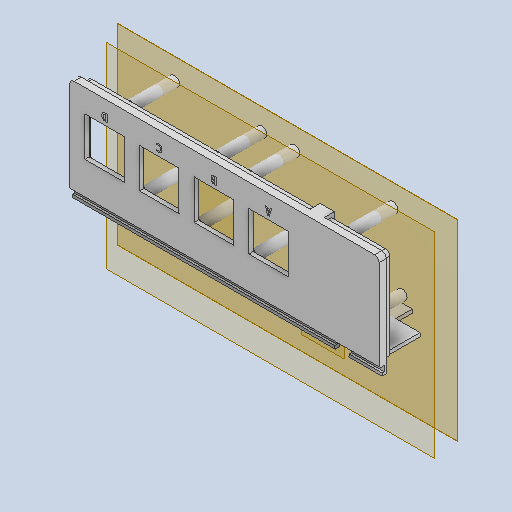
# Autodesk Inventor part: RV_ES_TopHV
Saved by Autodesk Inventor 2023.3 (Build 273359000, 359)
## iProperties
Created: 2023-08-06
Part Number: RV_ES_TopHV
Material: Generic
Document SubType Name: Modeling
Designer: atrus
Density: 1 g/cm^3
Appearance: Default
Author: atrus
Autodesk Inventor part; units mm, degrees
ref_plane "YZ Plane" through (0, 0, 0) normal (1, 0, 0) x (0, 1, 0)
ref_plane "XZ Plane" through (0, 0, 0) normal (0, 1, 0) x (-1, 0, 0)
ref_plane "XY Plane" through (0, 0, 0) normal (0, 0, 1) x (1, 0, 0)
ref_plane "Work Plane1" through (160.7185, -7.9424, -39.0916) normal (0, 0, 1) x (1, 0, 0)
ref_plane "Bottom Case Offset" through (160.7185, -7.9424, -38.8916) normal (0, 0, 1) x (1, 0, 0)
sketch "Sketch1" plane through (0, 0, 0) normal (0, 0, 1) x (1, 0, 0)
  line L0 (0, 55.6141) -> (215.9, 55.6141)
  line L1 (215.9, 55.6141) -> (215.9, 121.7246)
  line L2 (215.9, 121.7246) -> (0, 121.7246)
  line L3 (0, 121.7246) -> (0, 55.6141)
  line L4 (215.9, 121.7246) -> (215.9, 57.6563) construction
  line L5 (19.0355, 55.6141) -> (3.81, 55.6141) construction
  line L6 (0, 48.8987) -> (0, 118.5496) construction
  point P0 (0, 88.6694)
  constraints: 8 end point, 2 horizontal, 1 collinear, 1 midpoint, 1 parallel, 1 perpendicular, 1 point on line, 3 other
extrude "Top Face" add sketch "Sketch1" along normal blind 5
sketch "Sketch2" plane through (0, 0, 5) normal (0, 0, 1) x (1, 0, 0)
  line L0 (37.1761, 79.276) -> (11.6745, 79.276) construction
  line L1 (37.1761, 104.7776) -> (37.1761, 79.276) construction
  line L2 (11.6745, 104.7776) -> (37.1761, 104.7776) construction
  line L3 (11.6745, 79.276) -> (11.6745, 104.7776) construction
  line L4 (49.7745, 79.276) -> (49.7745, 104.7776) construction
  line L5 (49.7745, 104.7776) -> (75.2761, 104.7776) construction
  line L6 (75.2761, 104.7776) -> (75.2761, 79.276) construction
  line L7 (75.2761, 79.276) -> (49.7745, 79.276) construction
  line L8 (87.8745, 79.276) -> (87.8745, 104.7776) construction
  line L9 (87.8745, 104.7776) -> (113.3761, 104.7776) construction
  line L10 (113.3761, 104.7776) -> (113.3761, 79.276) construction
  line L11 (113.3761, 79.276) -> (87.8745, 79.276) construction
  line L12 (125.9745, 79.276) -> (125.9745, 104.7776) construction
  line L13 (125.9745, 104.7776) -> (151.4761, 104.7776) construction
  line L14 (151.4761, 104.7776) -> (151.4761, 79.276) construction
  line L15 (151.4761, 79.276) -> (125.9745, 79.276) construction
  line L16 (38.1761, 78.276) -> (10.6745, 78.276)
  line L17 (10.6745, 78.276) -> (10.6745, 105.7776)
  line L18 (10.6745, 105.7776) -> (38.1761, 105.7776)
  line L19 (38.1761, 105.7776) -> (38.1761, 78.276)
  line L20 (76.2761, 78.276) -> (76.2761, 105.7776)
  line L21 (76.2761, 105.7776) -> (48.7745, 105.7776)
  line L22 (48.7745, 105.7776) -> (48.7745, 78.276)
  line L23 (48.7745, 78.276) -> (76.2761, 78.276)
  line L24 (114.3761, 78.276) -> (114.3761, 105.7776)
  line L25 (114.3761, 105.7776) -> (86.8745, 105.7776)
  line L26 (86.8745, 105.7776) -> (86.8745, 78.276)
  line L27 (86.8745, 78.276) -> (114.3761, 78.276)
  line L28 (152.4761, 78.276) -> (152.4761, 105.7776)
  line L29 (152.4761, 105.7776) -> (124.9745, 105.7776)
  line L30 (124.9745, 105.7776) -> (124.9745, 78.276)
  line L31 (124.9745, 78.276) -> (152.4761, 78.276)
  point P0 (0, 0)
  dimension "d2" = 1
  constraints: 32 end point, 3 collinear, 12 other
  measures "d2" distance between parallel lines of L19 L1
extrude "Recept Cutouts" cut sketch "Sketch2" against normal blind 3
sketch "Sketch3" plane through (0, 0, 0) normal (0, 0, -1) x (-1, 0, 0)
  circle A0 centre (-29.21, 112.8346) radius 3.75 construction
  circle A1 centre (-43.18, 69.6546) radius 3.75 construction
  circle A2 centre (-90.17, 112.8346) radius 3.75 construction
  circle A3 centre (-113.03, 112.8346) radius 3.75 construction
  circle A4 centre (-181.61, 112.8346) radius 3.75 construction
  circle A5 centre (-81.28, 69.6546) radius 3.75 construction
  circle A6 centre (-119.38, 69.6546) radius 3.75 construction
  circle A7 centre (-187.96, 63.3046) radius 3.75 construction
  circle A8 centre (-29.21, 112.8346) radius 3.55
  circle A9 centre (-43.18, 69.6546) radius 3.55
  circle A10 centre (-81.28, 69.6546) radius 3.55
  circle A11 centre (-90.17, 112.8346) radius 3.55
  circle A12 centre (-113.03, 112.8346) radius 3.55
  circle A13 centre (-119.38, 69.6546) radius 3.55
  circle A14 centre (-181.61, 112.8346) radius 3.55
  circle A15 centre (-187.96, 63.3046) radius 3.55
  point P0 (0, 0)
  dimension "d5" = 0.2
  constraints: 8 centre point, 7 equal radius
  measures "d5" radial gap between concentric circles of A4 A14
extrude "Bosses" add sketch "Sketch3" along normal up to surface (38.8916 mm away)
ref_plane "PCB Plane Offset" through (103.0168, 55.1564, -27.3288) normal (0, 0, 1) x (1, 0, 0)
sketch "Sketch4" plane through (0, 0, 0) normal (0, 0, -1) x (-1, 0, 0)
  line L0 (-172.95, 55.3986) -> (-195.35, 55.3986) construction
  line L1 (-195.35, 58.3986) -> (-172.95, 58.3986) construction
  line L2 (-182.51, 43.0986) -> (-182.51, 95.4986) construction
  line L3 (-183.01, 55.5986) -> (-212.09, 55.5986)
  line L4 (-212.09, 55.5986) -> (-212.09, 58.1986)
  line L5 (-212.09, 58.1986) -> (-183.01, 58.1986)
  line L6 (-183.01, 58.1986) -> (-183.01, 55.5986)
  line L7 (-212.09, 115.3746) -> (-212.09, -4.0054) construction
  point P0 (0, 0)
  point P1 (-212.09, 55.6846)
  dimension "d8" = 0.5
  dimension "d9" = 0.2
  dimension "d10" = 0.2
  constraints: 8 end point, 3 perpendicular, 1 horizontal, 1 midpoint, 1 point on line
  measures "d8" distance between parallel lines of L2 L6
  measures "d9" distance between parallel lines of L0 L3
  measures "d10" distance between parallel lines of L1 L5
extrude "PS Side Tall Barrier" add sketch "Sketch4" along normal up to surface (27.3288 mm away)
sketch "Sketch5" plane through (212.09, 58.1986, -27.3288) normal (0, 0, -1) x (-1, 0, 0)
  line L0 (29.08, 0) -> (29.08, -2.5845) projected
  line L1 (29.08, 0) -> (0, 0) projected
  line L2 (29.08, -2.5845) -> (16.94, -2.5845)
  line L3 (16.94, -2.5845) -> (16.94, 0)
  line L4 (16.94, 0) -> (29.08, 0)
  line L5 (29.08, 0) -> (29.08, -2.5845)
  point P0 (212.09, -58.1986)
  point P1 (16.74, -2.8)
  dimension "d13" = 0.2
  constraints: 8 end point, 2 parallel, 1 horizontal, 1 perpendicular, 1 point on line, 1 other
  measures "d13" horizontal distance of point (16.74, -2.8) L2.end
extrude "PS Side Tall Barrier PCB" add sketch "Sketch5" along normal up to surface (11.5628 mm away)
sketch "Sketch6" plane through (0, 0, 0) normal (0, 0, -1) x (-1, 0, 0)
  arc A0 (-212.725, 121.7246) -> (-215.9, 118.5496) centre (-212.725, 118.5496) ccw construction
  arc A1 (-210.312, 119.3116) -> (-213.487, 116.1366) centre (-210.312, 116.1366) ccw construction
  line L0 (-213.487, 50.8987) -> (-213.487, 116.1366) construction
  line L1 (-210.312, 119.3116) -> (-172.72, 119.3116) construction
  line L2 (-162.72, 119.3116) -> (-5.588, 119.3116) construction
  arc A2 (-2.413, 116.1366) -> (-5.588, 119.3116) centre (-5.588, 116.1366) ccw construction
  line L3 (-2.413, 116.1366) -> (-2.413, 57.6563) construction
  line L4 (-213.287, 56.1141) -> (-213.287, 116.1366)
  arc A3 (-210.312, 119.1116) -> (-213.287, 116.1366) centre (-210.312, 116.1366) ccw
  line L5 (-210.312, 119.1116) -> (-172.72, 119.1116)
  line L6 (-162.72, 119.1116) -> (-5.588, 119.1116)
  arc A4 (-2.613, 116.1366) -> (-5.588, 119.1116) centre (-5.588, 116.1366) ccw
  line L7 (-2.613, 116.1366) -> (-2.613, 57.6563)
  line L8 (-211.287, 56.1141) -> (-211.287, 116.1366)
  arc A5 (-210.312, 117.1116) -> (-211.287, 116.1366) centre (-210.312, 116.1366) ccw
  arc A6 (-4.613, 116.1366) -> (-5.588, 117.1116) centre (-5.588, 116.1366) ccw
  line L9 (-4.613, 116.1366) -> (-4.613, 57.6563)
  line L10 (-211.287, 56.1141) -> (-213.287, 56.1141)
  line L11 (-4.613, 57.6563) -> (-2.613, 57.6563)
  line L12 (-162.72, 119.1116) -> (-162.72, 117.1116)
  line L13 (-172.72, 117.1116) -> (-172.72, 119.1116)
  circle A7 centre (-181.61, 112.8346) radius 3.55
  line L14 (-178.06, 112.8346) -> (-178.06, 117.1116)
  circle A8 centre (-113.03, 112.8346) radius 3.55
  line L15 (-116.58, 112.8346) -> (-116.58, 117.1116)
  line L16 (-109.48, 112.8346) -> (-109.48, 117.1116)
  circle A9 centre (-90.17, 112.8346) radius 3.55
  line L17 (-93.72, 112.8346) -> (-93.72, 117.1116)
  line L18 (-86.62, 112.8346) -> (-86.62, 117.1116)
  circle A10 centre (-29.21, 112.8346) radius 3.55
  line L19 (-32.76, 112.8346) -> (-32.76, 117.1116)
  line L20 (-25.66, 112.8346) -> (-25.66, 117.1116)
  circle A11 centre (-181.61, 112.8346) radius 3.55
  circle A12 centre (-113.03, 112.8346) radius 3.55
  line L21 (-185.16, 112.8346) -> (-185.16, 117.1116)
  line L22 (-210.312, 117.1116) -> (-185.16, 117.1116)
  line L23 (-178.06, 117.1116) -> (-172.72, 117.1116)
  line L24 (-162.72, 117.1116) -> (-116.58, 117.1116)
  line L25 (-109.48, 117.1116) -> (-93.72, 117.1116)
  line L26 (-86.62, 117.1116) -> (-32.76, 117.1116)
  line L27 (-25.66, 117.1116) -> (-5.588, 117.1116)
extrude "Inner Lip" add sketch "Sketch6" along normal blind 5 contours L4 A3 L5 L13 L23 L14 A7 L21 L22 A5 L8 L10 | L6 A4 L7 L11 L9 A6 L27 L20 A10 L19 L26 L18 A9 L17 L25 L16 A8 L15 L24 L12
sketch "Sketch7" plane through (181.61, 112.8346, -38.8916) normal (0, 0, -1) x (-1, 0, 0)
  circle A0 centre (0, 0) radius 3.55 projected
  circle A1 centre (68.58, 0) radius 3.55 projected
  circle A2 centre (91.44, 0) radius 3.55 projected
  circle A3 centre (152.4, 0) radius 3.55 projected
  circle A4 centre (138.43, -43.18) radius 3.55 projected
  circle A5 centre (100.33, -43.18) radius 3.55 projected
  circle A6 centre (62.23, -43.18) radius 3.55 projected
  circle A7 centre (-6.35, -49.53) radius 3.55 projected
  point P0 (181.61, -112.8346)
hole "Boss Holes" at (181.61, 112.8346, -38.8916) at (113.03, 112.8346, -38.8916) at (90.17, 112.8346, -38.8916) at (29.21, 112.8346, -38.8916) at (43.18, 69.6546, -38.8916) at (81.28, 69.6546, -38.8916) at (119.38, 69.6546, -38.8916) at (187.96, 63.3046, -38.8916) direction (0, 0, 1) diameter 2.1565 depth 12.7 tip angle 118 thread size "4-40 UNC" class "2B" standard "ANSI Unified Screw Threads"
sketch "Sketch8" plane through (0, 0, 0) normal (0, 0, -1) x (-1, 0, 0)
  line L0 (-162.72, 117.1116) -> (-162.72, 121.7246)
  line L1 (-215.9, 121.7246) -> (0, 121.7246) projected
  line L2 (-172.72, 117.1116) -> (-172.72, 121.7246)
  line L3 (-162.72, 117.1116) -> (-116.58, 117.1116) construction
  line L4 (-172.72, 117.1116) -> (-162.72, 117.1116)
  line L5 (-178.06, 117.1116) -> (-172.72, 117.1116) projected
  line L6 (-172.72, 117.1116) -> (-172.72, 119.1116) projected
  line L7 (-162.72, 119.1116) -> (-162.72, 117.1116) projected
  line L8 (-172.72, 121.7246) -> (-162.72, 121.7246)
  point P0 (0, 0)
  point P1 (-172.72, 118.1116)
  constraints: 8 end point, 3 collinear, 1 horizontal, 1 midpoint, 1 perpendicular, 1 point on line, 1 vertical
extrude "Cord Relief" add sketch "Sketch8" along normal blind 7
fillet "Boss Filets" radius 3.175 8 edges at (181.61, 109.2846, 0) (46.73, 69.6546, 0) (84.83, 69.6546, 0) (122.93, 69.6546, 0) (191.51, 63.3046, 0) (113.03, 109.2846, 0) (90.17, 109.2846, 0) (29.21, 109.2846, 0)
ref_plane "Relay Top" through (39.6501, 64.8987, -6.5239) normal (0, 0, 1) x (1, 0, 0)
ref_plane "PS Top" through (155.31, 43.0986, -2.5541) normal (0, 0, 1) x (0, 1, 0)
sketch "Sketch10" plane through (0, 0, 0) normal (0, 0, -1) x (-1, 0, 0)
  line L0 (-116.8501, 57.6563) -> (-122.4501, 57.6563) construction
  line L1 (-78.7501, 57.6563) -> (-84.3501, 57.6563) construction
  line L2 (-40.6501, 57.6563) -> (-46.2501, 57.6563) construction
  line L3 (-2.413, 57.6563) -> (-8.1501, 57.6563) construction
  line L4 (-153.9501, 48.8987) -> (-153.9501, 64.8987) construction
  line L5 (-155.31, 95.4986) -> (-155.31, 43.0986) construction
  line L6 (-182.51, 43.0986) -> (-182.51, 95.4986) construction
  line L7 (0, 55.6141) -> (-183.01, 55.6141)
  line L8 (-122.9501, 55.6141) -> (-153.4501, 55.6141)
  line L9 (-153.4501, 55.6141) -> (-153.4501, 57.6141)
  line L10 (-153.4501, 57.6141) -> (-122.9501, 57.6141)
  line L11 (-122.9501, 57.6141) -> (-122.9501, 55.6141)
  line L12 (-116.3501, 55.6141) -> (-84.8501, 55.6141)
  line L13 (-84.8501, 55.6141) -> (-84.8501, 57.6141)
  line L14 (-84.8501, 57.6141) -> (-116.3501, 57.6141)
  line L15 (-116.3501, 57.6141) -> (-116.3501, 55.6141)
  line L16 (-78.2421, 55.6141) -> (-46.7501, 55.6141)
  line L17 (-46.7501, 55.6141) -> (-46.7501, 57.6141)
  line L18 (-46.7501, 57.6141) -> (-78.2421, 57.6141)
  line L19 (-78.2421, 57.6141) -> (-78.2421, 55.6141)
  line L20 (-40.1501, 55.6141) -> (-8.6501, 55.6141)
  line L21 (-8.6501, 55.6141) -> (-8.6501, 57.6141)
  line L22 (-8.6501, 57.6141) -> (-40.1501, 57.6141)
  line L23 (-40.1501, 57.6141) -> (-40.1501, 55.6141)
  point P0 (0, 0)
  point P1 (-8.6501, 55.6141)
  point P2 (-78.2421, 55.6141)
  point P3 (-78.2421, 56.6141)
extrude "Barrier Relay" add sketch "Sketch10" along normal up to surface (6.5239 mm away)
sketch "Sketch11" plane through (0, 0, 0) normal (0, 0, -1) x (-1, 0, 0)
  line L0 (-155.31, 95.4986) -> (-155.31, 43.0986) construction
  line L1 (-182.51, 43.0986) -> (-182.51, 95.4986) construction
  line L2 (-153.9501, 48.8987) -> (-153.9501, 64.8987) construction
  line L3 (0, 55.6141) -> (-215.9, 55.6141) projected
  line L4 (-182.01, 55.6141) -> (-155.81, 55.6141)
  line L5 (-155.81, 55.6141) -> (-155.81, 57.6141)
  line L6 (-155.81, 57.6141) -> (-182.01, 57.6141)
  line L7 (-182.01, 57.6141) -> (-182.01, 55.6141)
  point P0 (0, 0)
  point P1 (-182.01, 56.6141)
  point P2 (-155.81, 56.6141)
  dimension "d55" = 0.5
  dimension "d56" = 0.5
  constraints: 8 end point, 2 midpoint, 2 parallel, 1 horizontal, 1 perpendicular, 1 point on line
  measures "d55" distance from line of L1 point (-182.01, 56.614)
  measures "d56" distance from line of point (-155.81, 56.614) L0
extrude "Barrier PSU" add sketch "Sketch11" along normal up to surface (2.5541 mm away)
fillet "Outside corner fillets" radius 3.175 2 edges at (215.9, 121.7246, 2.5) (0, 121.7246, 2.5)
fillet "Outer Boss Fillets" radius 3.175 4 edges at (29.21, 116.3846, -5) (90.17, 116.3846, -5) (113.03, 116.3846, -5) (181.61, 116.3846, -5)
ref_plane "TopReceptSeatOffset" through (100.6253, 92.0268, 2.44) normal (0, 0, 1) x (-1, 0, 0)
sketch "Sketch12" plane through (0, 0, 0) normal (0, 0, -1) x (-1, 0, 0)
  line L0 (-12.8302, 76.4693) -> (-36.0204, 76.4693) construction
  arc A0 (-12.8302, 76.4693) -> (-8.8678, 80.4317) centre (-12.8302, 80.4317) ccw construction
  line L1 (-8.8678, 103.6219) -> (-8.8678, 80.4317) construction
  arc A1 (-8.8678, 103.6219) -> (-12.8302, 107.5843) centre (-12.8302, 103.6219) ccw construction
  line L2 (-36.0204, 107.5843) -> (-12.8302, 107.5843) construction
  arc A2 (-36.0204, 107.5843) -> (-39.9828, 103.6219) centre (-36.0204, 103.6219) ccw construction
  line L3 (-39.9828, 80.4317) -> (-39.9828, 103.6219) construction
  arc A3 (-39.9828, 80.4317) -> (-36.0204, 76.4693) centre (-36.0204, 80.4317) ccw construction
  line L4 (-35.5886, 80.0761) -> (-13.2366, 80.0761) construction
  arc A4 (-36.3506, 80.8381) -> (-35.5886, 80.0761) centre (-35.5886, 80.8381) ccw construction
  line L5 (-36.3506, 93.7921) -> (-36.3506, 80.8381) construction
  arc A5 (-35.5886, 94.5541) -> (-36.3506, 93.7921) centre (-35.5886, 93.7921) ccw construction
  line L6 (-32.8073, 94.5541) -> (-35.5886, 94.5541) construction
  arc A6 (-32.8073, 94.5541) -> (-32.0453, 95.3161) centre (-32.8073, 95.3161) ccw construction
  line L7 (-32.0453, 103.1901) -> (-32.0453, 95.3161) construction
  arc A7 (-31.2833, 103.9521) -> (-32.0453, 103.1901) centre (-31.2833, 103.1901) ccw construction
  line L8 (-17.5673, 103.9521) -> (-31.2833, 103.9521) construction
  arc A8 (-16.8053, 103.1901) -> (-17.5673, 103.9521) centre (-17.5673, 103.1901) ccw construction
  line L9 (-16.8053, 95.3161) -> (-16.8053, 103.1901) construction
  arc A9 (-16.8053, 95.3161) -> (-16.0433, 94.5541) centre (-16.0433, 95.3161) ccw construction
  line L10 (-13.2366, 94.5541) -> (-16.0433, 94.5541) construction
  arc A10 (-12.4746, 93.7921) -> (-13.2366, 94.5541) centre (-13.2366, 93.7921) ccw construction
  line L11 (-12.4746, 80.8381) -> (-12.4746, 93.7921) construction
  arc A11 (-13.2366, 80.0761) -> (-12.4746, 80.8381) centre (-13.2366, 80.8381) ccw construction
  line L12 (-50.9302, 76.4693) -> (-74.1204, 76.4693) construction
  arc A12 (-50.9302, 76.4693) -> (-46.9678, 80.4317) centre (-50.9302, 80.4317) ccw construction
  line L13 (-46.9678, 103.6219) -> (-46.9678, 80.4317) construction
  arc A13 (-46.9678, 103.6219) -> (-50.9302, 107.5843) centre (-50.9302, 103.6219) ccw construction
  line L14 (-74.1204, 107.5843) -> (-50.9302, 107.5843) construction
  arc A14 (-74.1204, 107.5843) -> (-78.0828, 103.6219) centre (-74.1204, 103.6219) ccw construction
  line L15 (-78.0828, 80.4317) -> (-78.0828, 103.6219) construction
  arc A15 (-78.0828, 80.4317) -> (-74.1204, 76.4693) centre (-74.1204, 80.4317) ccw construction
  line L16 (-73.6886, 80.0761) -> (-51.3366, 80.0761) construction
  arc A16 (-74.4506, 80.8381) -> (-73.6886, 80.0761) centre (-73.6886, 80.8381) ccw construction
  line L17 (-74.4506, 93.7921) -> (-74.4506, 80.8381) construction
  arc A17 (-73.6886, 94.5541) -> (-74.4506, 93.7921) centre (-73.6886, 93.7921) ccw construction
  line L18 (-70.9073, 94.5541) -> (-73.6886, 94.5541) construction
  arc A18 (-70.9073, 94.5541) -> (-70.1453, 95.3161) centre (-70.9073, 95.3161) ccw construction
  line L19 (-70.1453, 103.1901) -> (-70.1453, 95.3161) construction
  arc A19 (-69.3833, 103.9521) -> (-70.1453, 103.1901) centre (-69.3833, 103.1901) ccw construction
  line L20 (-55.6673, 103.9521) -> (-69.3833, 103.9521) construction
  arc A20 (-54.9053, 103.1901) -> (-55.6673, 103.9521) centre (-55.6673, 103.1901) ccw construction
  line L21 (-54.9053, 95.3161) -> (-54.9053, 103.1901) construction
  arc A21 (-54.9053, 95.3161) -> (-54.1433, 94.5541) centre (-54.1433, 95.3161) ccw construction
  line L22 (-51.3366, 94.5541) -> (-54.1433, 94.5541) construction
  arc A22 (-50.5746, 93.7921) -> (-51.3366, 94.5541) centre (-51.3366, 93.7921) ccw construction
  line L23 (-50.5746, 80.8381) -> (-50.5746, 93.7921) construction
  arc A23 (-51.3366, 80.0761) -> (-50.5746, 80.8381) centre (-51.3366, 80.8381) ccw construction
  line L24 (-116.1828, 80.4317) -> (-116.1828, 103.6219) construction
  arc A24 (-112.2204, 107.5843) -> (-116.1828, 103.6219) centre (-112.2204, 103.6219) ccw construction
  line L25 (-112.2204, 107.5843) -> (-89.0302, 107.5843) construction
  arc A25 (-85.0678, 103.6219) -> (-89.0302, 107.5843) centre (-89.0302, 103.6219) ccw construction
  line L26 (-85.0678, 103.6219) -> (-85.0678, 80.4317) construction
  arc A26 (-89.0302, 76.4693) -> (-85.0678, 80.4317) centre (-89.0302, 80.4317) ccw construction
  line L27 (-89.0302, 76.4693) -> (-112.2204, 76.4693) construction
  arc A27 (-116.1828, 80.4317) -> (-112.2204, 76.4693) centre (-112.2204, 80.4317) ccw construction
  line L28 (-87.8745, 79.276) -> (-113.3761, 79.276) construction
  line L29 (-87.8745, 104.7776) -> (-87.8745, 79.276) construction
  line L30 (-113.3761, 104.7776) -> (-87.8745, 104.7776) construction
  line L31 (-113.3761, 79.276) -> (-113.3761, 104.7776) construction
  line L32 (-127.1302, 76.4693) -> (-150.3204, 76.4693) construction
  arc A28 (-127.1302, 76.4693) -> (-123.1678, 80.4317) centre (-127.1302, 80.4317) ccw construction
  line L33 (-123.1678, 103.6219) -> (-123.1678, 80.4317) construction
  arc A29 (-123.1678, 103.6219) -> (-127.1302, 107.5843) centre (-127.1302, 103.6219) ccw construction
  line L34 (-150.3204, 107.5843) -> (-127.1302, 107.5843) construction
  arc A30 (-150.3204, 107.5843) -> (-154.2828, 103.6219) centre (-150.3204, 103.6219) ccw construction
  line L35 (-154.2828, 80.4317) -> (-154.2828, 103.6219) construction
  arc A31 (-154.2828, 80.4317) -> (-150.3204, 76.4693) centre (-150.3204, 80.4317) ccw construction
  arc A32 (-36.0204, 108.5843) -> (-40.9828, 103.6219) centre (-36.0204, 103.6219) ccw
  line L36 (-36.0204, 108.5843) -> (-12.8302, 108.5843)
  arc A33 (-7.8678, 103.6219) -> (-12.8302, 108.5843) centre (-12.8302, 103.6219) ccw
  line L37 (-7.8678, 103.6219) -> (-7.8678, 80.4317)
  arc A34 (-12.8302, 75.4693) -> (-7.8678, 80.4317) centre (-12.8302, 80.4317) ccw
  line L38 (-12.8302, 75.4693) -> (-36.0204, 75.4693)
  arc A35 (-40.9828, 80.4317) -> (-36.0204, 75.4693) centre (-36.0204, 80.4317) ccw
  line L39 (-40.9828, 80.4317) -> (-40.9828, 103.6219)
  arc A36 (-50.9302, 75.2448) -> (-45.7434, 80.4317) centre (-50.9302, 80.4317) ccw
  line L40 (-50.9302, 75.2448) -> (-74.1204, 75.2448)
  arc A37 (-79.3073, 80.4317) -> (-74.1204, 75.2448) centre (-74.1204, 80.4317) ccw
  line L41 (-79.3073, 80.4317) -> (-79.3073, 103.6219)
  arc A38 (-74.1204, 108.8087) -> (-79.3073, 103.6219) centre (-74.1204, 103.6219) ccw
  line L42 (-74.1204, 108.8087) -> (-50.9302, 108.8087)
  arc A39 (-45.7434, 103.6219) -> (-50.9302, 108.8087) centre (-50.9302, 103.6219) ccw
  line L43 (-45.7434, 103.6219) -> (-45.7434, 80.4317)
  line L44 (-83.9929, 80.4317) -> (-83.9929, 103.6219)
  arc A40 (-83.9929, 103.6219) -> (-89.0302, 108.6592) centre (-89.0302, 103.6219) ccw
  line L45 (-89.0302, 108.6592) -> (-112.2204, 108.6592)
  arc A41 (-112.2204, 108.6592) -> (-117.2578, 103.6219) centre (-112.2204, 103.6219) ccw
  line L46 (-117.2578, 103.6219) -> (-117.2578, 80.4317)
  arc A42 (-117.2578, 80.4317) -> (-112.2204, 75.3943) centre (-112.2204, 80.4317) ccw
  line L47 (-112.2204, 75.3943) -> (-89.0302, 75.3943)
  arc A43 (-89.0302, 75.3943) -> (-83.9929, 80.4317) centre (-89.0302, 80.4317) ccw
  arc A44 (-127.1302, 75.6094) -> (-122.3079, 80.4317) centre (-127.1302, 80.4317) ccw
  line L48 (-127.1302, 75.6094) -> (-150.3204, 75.6094)
  arc A45 (-155.1427, 80.4317) -> (-150.3204, 75.6094) centre (-150.3204, 80.4317) ccw
  line L49 (-155.1427, 80.4317) -> (-155.1427, 103.6219)
  arc A46 (-150.3204, 108.4441) -> (-155.1427, 103.6219) centre (-150.3204, 103.6219) ccw
  line L50 (-150.3204, 108.4441) -> (-127.1302, 108.4441)
  arc A47 (-122.3079, 103.6219) -> (-127.1302, 108.4441) centre (-127.1302, 103.6219) ccw
  line L51 (-122.3079, 103.6219) -> (-122.3079, 80.4317)
  point P0 (0, 0)
  dimension "d66" = 1
  constraints: 32 end point, 32 point on circle, 16 centre point, 3 parallel, 28 other
  measures "d66" distance between parallel lines of L38 L0
extrude "Recept Inset" cut sketch "Sketch12" along normal blind 4 and the other way blind 2.0066
sketch "Sketch13" plane through (0, 55.6141, 0) normal (-1, 0, 0) x (0, 0, 1)
  line L0 (0, 0) -> (-6.5239, 0) projected
  line L1 (0, 0) -> (5, 0) projected
  line L2 (0, 0) -> (5, 0)
  line L3 (0, -6.7154) -> (0, 0)
  line L4 (0, 62.9355) -> (0, 0) projected
  line L5 (5, 0) -> (5, 62.9355) projected
  line L6 (5, 0) -> (5, 0)
  line L7 (4, -1) -> (1.5, -1)
  line L8 (1.5, -1) -> (1.5, -4.7154)
  line L9 (1.5, -4.7154) -> (3, -4.7154)
  line L10 (3, -4.7154) -> (3, -6.7154)
  line L11 (3, -6.7154) -> (0, -6.7154)
  line L12 (5, 0) -> (4, -1)
  line L13 (-23.8516, -6.7154) -> (-0.1, -6.7154) construction
  point P0 (0, -55.6141)
  point P1 (5, -1)
  point P2 (0, -3.3577)
  dimension "d73" = 2
  dimension "d74" = 1.5
  dimension "d75" = 1
  dimension "d76" = 2
  dimension "d77" = 1
  dimension "d78" = 1
  constraints: 18 end point, 5 perpendicular, 3 collinear, 2 point on line, 1 midpoint, 1 vertical
  measures "d73" distance between parallel lines of L6 L10
  measures "d74" distance from line of point (0, -3.358) L8
  measures "d75" distance of L1.end point (5, -1)
  measures "d76" distance of L9.end L10.end
  measures "d77" distance of L6.end point (5, -1)
  measures "d78" distance of L7.start point (5, -1)
extrude "TopFace Interlock" add sketch "Sketch13" against normal up to surface (215.9 mm away)
sketch "Sketch14" plane through (0, 0, 5) normal (0, 0, 1) x (1, 0, 0)
  line L0 (10.6745, 105.7776) -> (38.1761, 105.7776) construction
  line L1 (48.7745, 105.7776) -> (76.2761, 105.7776) construction
  line L2 (86.8745, 105.7776) -> (114.3761, 105.7776) construction
  line L3 (124.9745, 105.7776) -> (152.4761, 105.7776) construction
  line L4 (10.6745, 113.3976) -> (38.1761, 113.3976) construction
  line L5 (48.7745, 113.3976) -> (76.2761, 113.3976) construction
  line L6 (86.8745, 113.3976) -> (114.3761, 113.3976) construction
  line L7 (124.9745, 113.3976) -> (152.4761, 113.3976) construction
  line L8 (137.6101, 113.3976) -> (137.8878, 112.3961)
  line L9 (137.8878, 112.3961) -> (139.663, 112.3961)
  line L10 (139.663, 112.3961) -> (139.9498, 113.3976)
  line L11 (139.9498, 113.3976) -> (140.8966, 113.3976)
  line L12 (140.8966, 113.3976) -> (139.3945, 108.3176)
  line L13 (139.3945, 108.3176) -> (138.0562, 108.3176)
  line L14 (138.0562, 108.3176) -> (136.5495, 113.3976)
  line L15 (136.5495, 113.3976) -> (137.6101, 113.3976)
  line L16 (138.7618, 109.2462) -> (139.4354, 111.6132)
  line L17 (139.4354, 111.6132) -> (138.1063, 111.6132)
  line L18 (138.1063, 111.6132) -> (138.7618, 109.2462)
  line L19 (102.3141, 113.3976) -> (102.3141, 108.3176)
  line L20 (102.3141, 108.3176) -> (100.6754, 108.3176)
  spline S0 degree 2 poles (100.6754, 108.3176) (99.806, 108.3176) (98.9411, 108.923) (98.9411, 109.5375) knots 0 0 0 1 2 2 2
  spline S1 degree 2 poles (98.9411, 109.5375) (98.9411, 109.7241) (99.0321, 110.0883) (99.2188, 110.3887) (99.4964, 110.6209) (99.6876, 110.6891) knots 0 0 0 1 2 3 4 4 4
  spline S2 degree 2 poles (99.6876, 110.6891) (99.4964, 110.721) (99.1505, 110.9031) (98.891, 111.1944) (98.7408, 111.5904) (98.7408, 111.8362) knots 0 0 0 1 2 3 4 4 4
  spline S3 degree 2 poles (98.7408, 111.8362) (98.7408, 112.6146) (99.7832, 113.3976) (100.7664, 113.3976) knots 0 0 0 1 2 2 2
  line L21 (100.7664, 113.3976) -> (102.3141, 113.3976)
  spline S4 degree 2 poles (100.6982, 112.6146) (100.4706, 112.6146) (100.1246, 112.4963) (99.8879, 112.2914) (99.7696, 112.0138) (99.7696, 111.8544) knots 0 0 0 1 2 3 4 4 4
  spline S5 degree 2 poles (99.7696, 111.8544) (99.7696, 111.5221) (100.2612, 111.1489) (100.771, 111.1489) knots 0 0 0 1 2 2 2
  line L22 (100.771, 111.1489) -> (101.3673, 111.1489)
  line L23 (101.3673, 111.1489) -> (101.3673, 112.6146)
  line L24 (101.3673, 112.6146) -> (100.6982, 112.6146)
  spline S6 degree 2 poles (99.938, 109.7059) (99.938, 109.5602) (100.029, 109.3281) (100.2384, 109.1688) (100.5616, 109.0777) (100.7892, 109.0777) knots 0 0 0 1 2 3 4 4 4
  line L25 (100.7892, 109.0777) -> (101.3673, 109.0777)
  line L26 (101.3673, 109.0777) -> (101.3673, 110.416)
  line L27 (101.3673, 110.416) -> (100.7892, 110.416)
  spline S7 degree 2 poles (100.7892, 110.416) (100.5571, 110.416) (100.2339, 110.3022) (100.029, 110.1065) (99.938, 109.8516) (99.938, 109.7059) knots 0 0 0 1 2 3 4 4 4
  spline S8 degree 2 poles (60.8138, 113.1927) (61.1506, 113.3293) (61.7834, 113.4658) (62.1293, 113.4658) knots 0 0 0 1 2 2 2
  spline S9 degree 2 poles (62.1293, 113.4658) (62.6756, 113.4658) (63.5177, 113.1426) (64.0958, 112.5054) (64.3962, 111.5631) (64.3962, 110.9349) knots 0 0 0 1 2 3 4 4 4
  spline S10 degree 2 poles (64.3962, 110.9349) (64.3962, 110.2931) (64.0685, 109.2962) (63.463, 108.6043) (62.5982, 108.2447) (62.0565, 108.2447) knots 0 0 0 1 2 3 4 4 4
  spline S11 degree 2 poles (62.0565, 108.2447) (61.8835, 108.2447) (61.574, 108.2584) (61.2781, 108.3039) (60.9777, 108.3722) (60.8138, 108.4268) knots 0 0 0 1 2 3 4 4 4
  line L28 (60.8138, 108.4268) -> (60.8138, 109.3736)
  spline S12 degree 2 poles (60.8138, 109.3736) (61.1415, 109.2188) (61.7424, 109.0868) (61.9882, 109.0868) knots 0 0 0 1 2 2 2
  spline S13 degree 2 poles (61.9882, 109.0868) (62.3478, 109.0868) (62.8576, 109.3463) (63.1899, 109.8197) (63.3447, 110.4661) (63.3447, 110.8576) knots 0 0 0 1 2 3 4 4 4
  spline S14 degree 2 poles (63.3447, 110.8576) (63.3447, 111.2672) (63.1854, 111.9182) (62.8531, 112.3688) (62.3296, 112.6055) (61.9746, 112.6055) knots 0 0 0 1 2 3 4 4 4
  spline S15 degree 2 poles (61.9746, 112.6055) (61.8471, 112.6055) (61.5467, 112.5554) (61.2417, 112.4735) (60.9413, 112.3597) (60.8138, 112.3005) knots 0 0 0 1 2 3 4 4 4
  line L29 (60.8138, 112.3005) -> (60.8138, 113.1927)
  spline S16 degree 2 poles (22.4498, 110.7938) (22.4498, 111.3856) (22.7411, 112.346) (23.3602, 113.0288) (24.3206, 113.3976) (24.9943, 113.3976) knots 0 0 0 1 2 3 4 4 4
  line L30 (24.9943, 113.3976) -> (26.2825, 113.3976)
  line L31 (26.2825, 113.3976) -> (26.2825, 108.3176)
  line L32 (26.2825, 108.3176) -> (24.7804, 108.3176)
  spline S17 degree 2 poles (24.7804, 108.3176) (24.1977, 108.3176) (23.3238, 108.6089) (22.7411, 109.2143) (22.4498, 110.1474) (22.4498, 110.7938) knots 0 0 0 1 2 3 4 4 4
  spline S18 degree 2 poles (23.474, 110.8576) (23.474, 110.4433) (23.606, 109.7969) (23.9201, 109.3509) (24.4481, 109.1187) (24.8396, 109.1187) knots 0 0 0 1 2 3 4 4 4
  line L33 (24.8396, 109.1187) -> (25.3266, 109.1187)
  line L34 (25.3266, 109.1187) -> (25.3266, 112.5964)
  line L35 (25.3266, 112.5964) -> (24.9078, 112.5964)
  spline S19 degree 2 poles (24.9078, 112.5964) (24.2023, 112.5964) (23.474, 111.7588) (23.474, 110.8576) knots 0 0 0 1 2 2 2
  point P0 (0, 0)
  dimension "d82" = 7.62
  constraints: 8 end point, 4 horizontal, 4 parallel, 3 collinear
  measures "d82" distance between parallel lines of L4 L0
extrude "Extrusion13" cut sketch "Sketch14" against normal blind 0.001
sketch "Sketch16" plane through (0, 0, 0) normal (0, 0, -1) x (-1, 0, 0)
  circle A0 centre (-187.96, 50.6046) radius 3.45 construction
  circle A1 centre (-187.96, 50.6046) radius 4.994
  line L0 (-212.09, 55.5986) -> (-183.01, 55.5986) projected
  point P0 (0, 0)
  constraints: 1 centre point, 1 coincident, 1 tangent
extrude "Extrusion14" cut sketch "Sketch16" against normal blind 25.4
equation "\"d78\" = d77"
body "Solid1"
